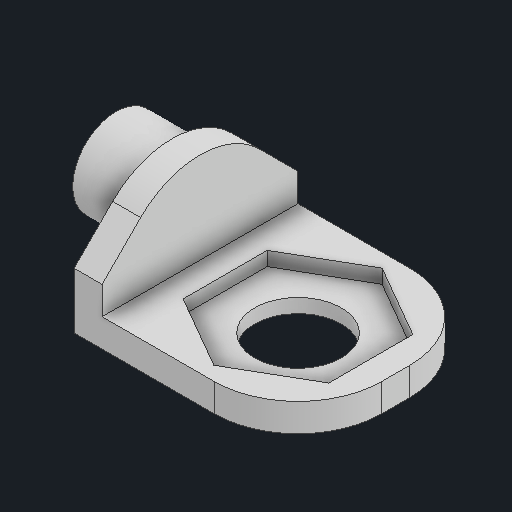
# Autodesk Inventor part: mocowanie_tofa_CPY1
Saved by Autodesk Inventor 2024 (Build 280153000, 153)
## iProperties
Created: 2024-05-24
Part Number: mocowanie_tofa_CPY1
Material: Generic
Document SubType Name: Modeling
Designer: Adam
Density: 1 g/cm^3
Appearance: Default
Author: Adam
Autodesk Inventor part; units mm, degrees
ref_plane "YZ Plane" through (0, 0, 0) normal (1, 0, 0) x (0, 1, 0)
ref_plane "XZ Plane" through (0, 0, 0) normal (0, 1, 0) x (-1, 0, 0)
ref_plane "XY Plane" through (0, 0, 0) normal (0, 0, 1) x (1, 0, 0)
sketch "Sketch1" plane through (0, 0, 0) normal (0, 0, 1) x (1, 0, 0)
  line L0 (0, 0) -> (8, 0)
  line L1 (8, 0) -> (8, 1)
  line L2 (8, 1) -> (1, 1)
  line L3 (1, 1) -> (1, 5)
  line L4 (1, 5) -> (0, 5)
  line L5 (0, 5) -> (0, 0)
  dimension "d0" = 8
  dimension "d1" = 5
  dimension "d2" = 1
  dimension "d8" = 1
  constraints: 12 end point, 5 perpendicular, 1 horizontal
  measures "d0" distance between parallel lines of L1 L5
  measures "d1" distance of L4.end L0.start
  measures "d2" distance between parallel lines of L2 L0
  measures "d8" distance between parallel lines of L3 L5
extrude "Extrusion1" add sketch "Sketch1" along normal blind 7
sketch "Sketch2" plane through (0, 0, 0) normal (-1, 0, 0) x (0, 0, 1)
  circle A0 centre (3.5, 2.55) radius 1.55
  line L0 (0, 0) -> (7, 0) projected
  line L1 (7, 5) -> (7, 0) projected
  dimension "d5" = 3.1
  dimension "d6" = 2.55
  dimension "d7" = 3.5
  constraints: 1 centre point
  measures "d5" diameter of A0
  measures "d6" distance from line of L0 A0.centre
  measures "d7" distance from line of L1 A0.centre
extrude "Extrusion2" add sketch "Sketch2" along normal blind 2
sketch "Sketch3" plane through (1, 1, 0) normal (0, 1, 0) x (1, 0, 0)
  line L0 (7, 0) -> (7, -7) projected
  line L1 (7, -7) -> (0, -7) projected
  point P0 (-1, 0)
  point P1 (3.5, -3.5)
  point P2 (3.5, -7)
  dimension "d11" = 3.5
  dimension "d12" = 3.5
  constraints: 1 midpoint
  measures "d11" distance from line of point (3.5, -3.5) L0
  measures "d12" distance of point (3.5, -7) point (3.5, -3.5)
hole "Hole1" at (4.5, 1, 3.5) direction (0, -1, 0) diameter 3.1 end through all
sketch "Sketch4" plane through (1, 1, 0) normal (0, 1, 0) x (1, 0, 0)
  line L0 (3.5, -0.495) -> (6.1024, -1.9975)
  line L1 (6.1024, -1.9975) -> (6.1024, -5.0025)
  line L2 (6.1024, -5.0025) -> (3.5, -6.505)
  line L3 (3.5, -6.505) -> (0.8976, -5.0025)
  line L4 (0.8976, -5.0025) -> (0.8976, -1.9975)
  line L5 (0.8976, -1.9975) -> (3.5, -0.495)
  circle A0 centre (3.5, -3.5) radius 1.55 projected
  point P0 (-1, 0)
  dimension "d20" = 6.01
  constraints: 12 end point, 3 coincident, 13 other
  measures "d20" distance of L0.start L2.end
fillet "Fillet1" radius 3 2 edges at (8, 0.5, 0) (8, 0.5, 7)
extrude "Extrusion3" cut sketch "Sketch4" against normal blind 0.5
chamfer "Chamfer1" distance 3 angle 45 2 edges at (0.5, 5, 7) (0.5, 5, 0)
fillet "Fillet2" radius 3 2 edges at (0.5, 5, 4) (0.5, 5, 3)
body "Solid1"
